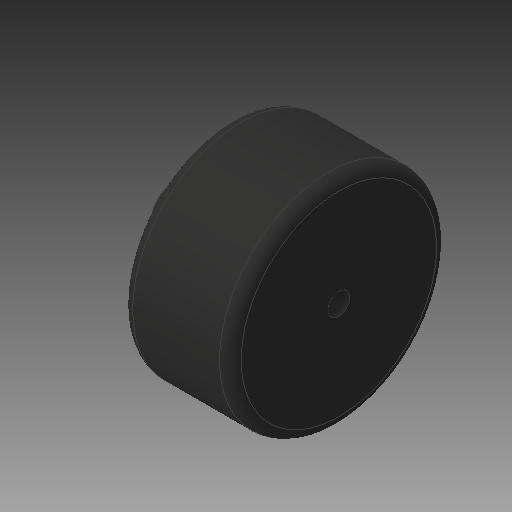
# Autodesk Inventor part: 100mm Mecanum StandIn
Saved by Autodesk Inventor 2019 (Build 230136000, 136)
## iProperties
Created: 2019-10-18
Part Number: 100mm Mecanum StandIn
Material: Rubber
Document SubType Name: Modeling
Designer: admin
Density: 0.93 g/cm^3
Appearance: Rubber - Black
Author: admin
Autodesk Inventor part; units mm, degrees
ref_plane "YZ Plane" through (0, 0, 0) normal (1, 0, 0) x (0, 1, 0)
ref_plane "XZ Plane" through (0, 0, 0) normal (0, 1, 0) x (-1, 0, 0)
ref_plane "XY Plane" through (0, 0, 0) normal (0, 0, 1) x (1, 0, 0)
sketch "Sketch1" plane through (0, 0, 0) normal (1, 0, 0) x (0, 1, 0)
  circle A0 centre (0, 0) radius 50
  dimension "d0" = 100
  constraints: 1 centre point, 1 coincident
  measures "d0" diameter of A0
extrude "Extrusion1" add sketch "Sketch1" along normal mid plane 50
fillet "Fillet1" radius 5 2 edges at (-25, -50, 0) (25, -50, 0)
sketch "Sketch3" plane through (-25, 0, 0) normal (-1, 0, 0) x (0, 0, 1)
  circle A0 centre (0, 0) radius 25
  dimension "d11" = 50
  constraints: 1 centre point, 1 coincident
  measures "d11" diameter of A0
extrude "Extrusion2" add sketch "Sketch3" along normal blind 5
sketch "Sketch4" plane through (-30, 0, 0) normal (-1, 0, 0) x (0, 0, 1)
  circle A0 centre (0, 0) radius 10
  dimension "d14" = 20
  constraints: 1 centre point, 1 coincident
  measures "d14" diameter of A0
extrude "Extrusion3" add sketch "Sketch4" along normal blind 21.4
sketch "Sketch5" plane through (-51.4, 0, 0) normal (-1, 0, 0) x (0, 0, 1)
  circle A0 centre (0, 0) radius 50 projected
  constraints: 1 coincident
hole "Hole2" at (-51.4, 0, 0) direction (1, 0, 0) diameter 10 end through all
sketch "Sketch6" plane through (0, 0, 0) normal (0, 1, 0) x (-1, 0, 0)
  circle A0 centre (41.2, 0) radius 3
  line L0 (51.4, -10) -> (51.4, 10) projected
  line L1 (41.2, 0) -> (51.4, 0) construction
  point P0 (0, 0)
  dimension "d24" = 6
  dimension "d25" = 10.2
  constraints: 2 end point, 1 centre point, 1 midpoint
  measures "d24" diameter of A0
  measures "d25" distance from line of L0 L1.start
extrude "Extrusion4" cut sketch "Sketch6" along normal blind 21.4
thread "Thread1" size "M6x1" class "6H" standard "ANSI Metric M Profile" full length
body "Solid1"
